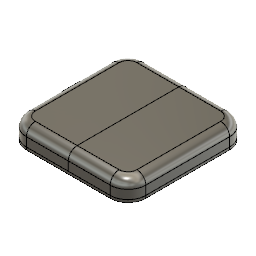
LightSwitch (Autodesk Fusion 360 design; units mm, degrees)
Autodesk Fusion 360 part; units mm, degrees
sketch "Sketch1" plane through (0, 0, 0) normal (0, 1, 0) x (1, 0, 0)
  line L0 (33.5, 33.5) -> (-33.5, -33.5) construction
  line L1 (-33.5, 33.5) -> (33.5, -33.5) construction
  line L2 (26.4289, -33.5) -> (33.5, -26.4289)
  line L3 (33.5, 26.4289) -> (26.4289, 33.5)
  line L4 (-26.4289, 33.5) -> (-33.5, 26.4289)
  line L5 (-33.5, -26.4289) -> (-26.4289, -33.5)
  line L6 (-33.5, 33.5) -> (-33.5, 26.4289)
  line L7 (-33.5, -26.4289) -> (-33.5, -33.5)
  line L8 (-33.5, 26.4289) -> (-33.5, -26.4289)
  line L9 (33.5, 33.5) -> (26.4289, 33.5)
  line L10 (-26.4289, 33.5) -> (-33.5, 33.5)
  line L11 (26.4289, 33.5) -> (-26.4289, 33.5)
  line L12 (-33.5, -33.5) -> (-26.4289, -33.5)
  line L13 (26.4289, -33.5) -> (33.5, -33.5)
  line L14 (-26.4289, -33.5) -> (26.4289, -33.5)
  line L15 (33.5, -33.5) -> (33.5, -26.4289)
  line L16 (33.5, 26.4289) -> (33.5, 33.5)
  line L17 (33.5, -26.4289) -> (33.5, 26.4289)
  line L18 (25.7919, 31.962) -> (-25.7919, 31.962)
  line L19 (-25.7919, 31.962) -> (-31.962, 25.7919)
  line L20 (-31.962, 25.7919) -> (-31.962, -25.7919)
  line L21 (-31.962, -25.7919) -> (-25.7919, -31.962)
  line L22 (-25.7919, -31.962) -> (25.7919, -31.962)
  line L23 (25.7919, -31.962) -> (31.962, -25.7919)
  line L24 (31.962, -25.7919) -> (31.962, 25.7919)
  line L25 (31.962, 25.7919) -> (25.7919, 31.962)
  dimension "d1" = 67
  dimension "d2" = 67
  dimension "d3" = 10
  dimension "d6" = 360
  dimension "d10" = 7.0711
  dimension "d11" = 1.538
extrude "Extrude1" add sketch "Sketch1" along normal blind 1.5 contours L2 L3 L4 L5 L8 L11 L14 L17 | L2 L13 L15 | L5 L7 L12 | L3 L9 L16 | L4 L6 L10 | L18 L19 L20 L21 L22 L23 L24 L25 makes body 1
extrude "Extrude2" add 1 faces at (8.8096, 1.5, 11.1667) along direction (0, 1, 0) blind 10 on bodies 1 bodies 1
delete_face "DeleteFace1" 1 faces at (-33.5, 3.8333, 28.786) on bodies 1
delete_face "DeleteFace2" 1 faces at (28.786, 3.8333, 33.5) on bodies 1
delete_face "DeleteFace3" 1 faces at (33.5, 3.8333, -28.786) on bodies 1
delete_face "DeleteFace4" 1 faces at (-28.786, 3.8333, -33.5) on bodies 1
fillet "Fillet1" radius 5 4 edges at (0, 11.5, 33.5) (-33.5, 11.5, 0) (0, 11.5, -33.5) (33.5, 11.5, 0) on bodies 1
fillet "Fillet1" radius 10 4 edges at (-33.5, 5.75, -33.5) (-33.5, 5.75, 33.5) (33.5, 5.75, 33.5) (33.5, 5.75, -33.5) on bodies 1
shell "Shell1" thickness 1.5 removed faces 0 bodies 1
ref_plane "WorkPlane1" through (29.9645, 1.5, -29.9645) normal (0, 1, 0) x (1, 0, 0)
split "Split1" by plane through (29.9645, 1.5, -29.9645) normal (0, 1, 0) bodies 1 makes body 2 at (7.8333, 11.5, 9.5)
sketch "Sketch3" plane through (0, 0, 0) normal (0, 0, 1) x (1, 0, 0)
  line L0 (31, 1.5) -> (31, 6.5)
  line L1 (32.5, 6.5) -> (25.4289, 6.5)
  line L2 (31, 1.5) -> (31, 3.5)
  line L3 (31, 3.5) -> (30, 3)
  line L4 (32.5, 1.5) -> (25.4289, 1.5)
  line L5 (31, 1.5) -> (29.9, 1.5)
  line L6 (29.4, 2) -> (29.4, 3.4501)
  line L7 (29.4, 3.4501) -> (29.4, 4)
  line L8 (29.4, 4) -> (30.5, 4)
  line L9 (30.5, 4) -> (29.4, 3.4501)
  line L10 (30, 2.5) -> (30, 3)
  line L11 (31, 1.5) -> (28.5, 1.5)
  line L12 (28.5, 4) -> (28.5, 2)
  arc A0 (29.4, 2) -> (29.9, 1.5) centre (29.9, 2) ccw
  line L13 (28, 1.5) -> (26.4, 1.5)
  arc A1 (28, 1.5) -> (28.5, 2) centre (28, 2) ccw
  line L14 (30, 2.5) -> (31, 1.7)
  line L15 (30.5, 4) -> (30.5, 4.5)
  line L16 (30.5, 4.5) -> (29.5, 5.5)
  line L17 (29.5, 5.5) -> (29, 5.5)
  line L18 (29, 5.5) -> (28.5, 4.5)
  line L19 (28.5, 4.5) -> (28.5, 4)
  dimension "d20" = 0.5
  dimension "d21" = 0.5
  measures "d20" radius of A0
  measures "d21" radius of A1
sketch "Tornillos" plane through (0, 0, 0) normal (0, 1, 0) x (1, 0, 0)
  line L0 (26.4289, 33.5) -> (-26.4289, 33.5)
  line L1 (-7.6716, 33.5) -> (8, 33.5)
  line L2 (0, 33.5) -> (0, 28.5)
  line L3 (1.75, 30) -> (-1.75, 30)
  line L4 (-3, 28.75) -> (-3, 28.25)
  line L5 (-1.75, 27) -> (1.75, 27)
  line L6 (3, 28.25) -> (3, 28.75)
  line L7 (10.2609, 33.6305) -> (-3, 27) construction
  line L8 (-3, 30) -> (3, 27) construction
  arc A0 (3, 28.75) -> (1.75, 30) centre (1.75, 28.75) ccw
  arc A1 (1.75, 27) -> (3, 28.25) centre (1.75, 28.25) ccw
  arc A2 (-3, 28.25) -> (-1.75, 27) centre (-1.75, 28.25) ccw
  arc A3 (-1.75, 30) -> (-3, 28.75) centre (-1.75, 28.75) ccw
  line L9 (0, 0) -> (9, 0)
  line L10 (-1.75, -27) -> (1.75, -27)
  arc A4 (-3, -28.75) -> (-1.75, -30) centre (-1.75, -28.75) ccw
  line L11 (-3, -28.75) -> (-3, -28.25)
  arc A5 (-1.75, -27) -> (-3, -28.25) centre (-1.75, -28.25) ccw
  line L12 (0, -33.5) -> (0, -28.5)
  line L13 (1.75, -30) -> (-1.75, -30)
  line L14 (3, -28.25) -> (3, -28.75)
  line L15 (-3, -30) -> (3, -27) construction
  arc A6 (1.75, -30) -> (3, -28.75) centre (1.75, -28.75) ccw
  arc A7 (3, -28.25) -> (1.75, -27) centre (1.75, -28.25) ccw
  line L16 (10.2609, -33.6305) -> (-3, -27) construction
  line L17 (33.5, -26.4289) -> (33.5, 26.4289)
  line L18 (33.5, -23.5) -> (33.5, 23.5)
  line L19 (32.5, 0) -> (25.4289, 0)
  line L20 (33.5, -7.15) -> (33.5, 7)
  line L21 (32.5, 0) -> (22.5, 0)
  circle A8 centre (22.5, 0) radius 1.75
  line L22 (0, 0) -> (0, 8)
  circle A9 centre (-22.5, 0) radius 1.75
  dimension "d33" = 6
  dimension "d34" = 3
  dimension "d35" = 1.25
  dimension "d36" = 5
  dimension "d37" = 3
  dimension "d38" = 10
  dimension "d39" = 3.5
  dimension "d43" = 4
  dimension "d44" = 10
  dimension "d45" = 3
  dimension "d46" = 3
  measures "d35" radius of A0
  measures "d37" distance of L3 L5
  measures "d39" diameter of A8
  measures "d44" distance of L11 L14
  measures "d45" distance of L10 L13
  measures "d46" distance of L14
extrude "Extrude7" cut sketch "Tornillos" along normal blind 10 contours L3 L4 L5 L6 A0 A1 A2 A3 | L10 A4 L11 A5 L13 L14 A6 A7 bodies 1
sketch "Sketch14" plane through (0, 1.5, 0) normal (0, 1, 0) x (-1, 0, 0)
  line L0 (1.75, -30) -> (-1.75, -30)
  arc A0 (-3, -28.75) -> (-1.75, -30) centre (-1.75, -28.75) ccw
  line L1 (-3, -28.75) -> (-3, -28.25)
  arc A1 (-1.75, -27) -> (-3, -28.25) centre (-1.75, -28.25) ccw
  line L2 (-1.75, -27) -> (1.75, -27)
  arc A2 (3, -28.25) -> (1.75, -27) centre (1.75, -28.25) ccw
  line L3 (3, -28.25) -> (3, -28.75)
  arc A3 (1.75, -30) -> (3, -28.75) centre (1.75, -28.75) ccw
  line L4 (-1.75, 30) -> (1.75, 30)
  arc A4 (3, 28.75) -> (1.75, 30) centre (1.75, 28.75) ccw
  line L5 (3, 28.75) -> (3, 28.25)
  arc A5 (1.75, 27) -> (3, 28.25) centre (1.75, 28.25) ccw
  line L6 (1.75, 27) -> (-1.75, 27)
  arc A6 (-3, 28.25) -> (-1.75, 27) centre (-1.75, 28.25) ccw
  line L7 (-3, 28.25) -> (-3, 28.75)
  arc A7 (-1.75, 30) -> (-3, 28.75) centre (-1.75, 28.75) ccw
  arc A8 (33.5, 23.5) -> (23.5, 33.5) centre (23.5, 23.5) ccw
  line L8 (23.5, 33.5) -> (-23.5, 33.5)
  arc A9 (-23.5, 33.5) -> (-33.5, 23.5) centre (-23.5, 23.5) ccw
  line L9 (-33.5, 23.5) -> (-33.5, -23.5)
  arc A10 (-33.5, -23.5) -> (-23.5, -33.5) centre (-23.5, -23.5) ccw
  line L10 (-23.5, -33.5) -> (23.5, -33.5)
  arc A11 (23.5, -33.5) -> (33.5, -23.5) centre (23.5, -23.5) ccw
  line L11 (33.5, -23.5) -> (33.5, 23.5)
  line L12 (33.5, -33.5) -> (-33.5, -33.5)
  line L13 (-1.75, 30) -> (1.75, 30)
  line L14 (1.75, 27) -> (-1.75, 27)
  line L15 (-3, 28.25) -> (-3, 28.75)
  line L16 (-33.5, 33.5) -> (33.5, 33.5)
  line L17 (33.5, 33.5) -> (33.5, -33.5)
  line L18 (3, 28.75) -> (3, 28.25)
  line L19 (-1.75, -27) -> (1.75, -27)
  line L20 (1.75, -30) -> (-1.75, -30)
  line L21 (-3, -28.75) -> (-3, -28.25)
  line L22 (30.9, -21) -> (29, -21)
  line L23 (30.9, 7.5) -> (29, 7.5)
  line L24 (-33.5, 33.5) -> (33.5, -33.5) construction
  line L25 (9.5, -22.5) -> (19.5, -22.5)
  line L26 (-9.5, -29.5) -> (-9.5, -22.5)
  line L27 (29, 7.5) -> (29, 21)
  line L28 (19.5, -29.5) -> (9.5, -29.5)
  line L29 (19.5, -22.5) -> (19.5, -29.5)
  line L30 (29, -21) -> (29, -7.5)
  line L31 (0, 0) -> (0, -4)
  line L32 (-19.5, -29.5) -> (-9.5, -29.5)
  line L33 (0, 0) -> (-9, 0)
  line L34 (-19.5, -22.5) -> (-19.5, -29.5)
  line L35 (29, -7.5) -> (30.9, -7.5)
  line L36 (-9.5, 22.5) -> (-19.5, 22.5)
  line L37 (-9.5, 29.5) -> (-9.5, 22.5)
  line L38 (-33.5, -33.5) -> (-33.5, 33.5)
  line L39 (30.9, -7.5) -> (30.9, -21)
  line L40 (33.5, 33.5) -> (-33.5, -33.5) construction
  line L41 (0, 0) -> (-4.5, 0)
  line L42 (-9.5, -22.5) -> (-19.5, -22.5)
  line L43 (9.5, -29.5) -> (9.5, -22.5)
  line L44 (-33.5, 23.5) -> (-33.5, -23.5)
  line L45 (-30.9, 21) -> (-29, 21)
  line L46 (33.5, -23.5) -> (33.5, 23.5)
  line L47 (-23.5, -33.5) -> (23.5, -33.5)
  line L48 (-19.5, 29.5) -> (-9.5, 29.5)
  arc A12 (1.75, 27) -> (3, 28.25) centre (1.75, 28.25) ccw
  arc A13 (-3, 28.25) -> (-1.75, 27) centre (-1.75, 28.25) ccw
  line L49 (19.5, 29.5) -> (9.5, 29.5)
  arc A14 (-3, -28.75) -> (-1.75, -30) centre (-1.75, -28.75) ccw
  line L50 (-30.9, 7.5) -> (-30.9, 21)
  line L51 (29, 21) -> (30.9, 21)
  arc A15 (1.75, -30) -> (3, -28.75) centre (1.75, -28.75) ccw
  arc A16 (3, 28.75) -> (1.75, 30) centre (1.75, 28.75) ccw
  arc A17 (-23.5, 33.5) -> (-33.5, 23.5) centre (-23.5, 23.5) ccw
  arc A18 (-33.5, -23.5) -> (-23.5, -33.5) centre (-23.5, -23.5) ccw
  arc A19 (-1.75, -27) -> (-3, -28.25) centre (-1.75, -28.25) ccw
  arc A20 (-1.75, 30) -> (-3, 28.75) centre (-1.75, 28.75) ccw
  arc A21 (3, -28.25) -> (1.75, -27) centre (1.75, -28.25) ccw
  arc A22 (23.5, -33.5) -> (33.5, -23.5) centre (23.5, -23.5) ccw
  line L52 (-19.5, 22.5) -> (-19.5, 29.5)
  line L53 (9.5, 22.5) -> (19.5, 22.5)
  circle A23 centre (22.5, 0) radius 1.75
  line L54 (9.5, 29.5) -> (9.5, 22.5)
  circle A24 centre (-22.5, 0) radius 1.75
  line L55 (19.5, 22.5) -> (19.5, 29.5)
  arc A25 (33.5, 23.5) -> (23.5, 33.5) centre (23.5, 23.5) ccw
  line L56 (30.9, 21) -> (30.9, 7.5)
  line L57 (23.5, 33.5) -> (-23.5, 33.5)
  line L58 (-29, -7.5) -> (-29, -21)
  line L59 (-29, -21) -> (-30.9, -21)
  line L60 (-29, 7.5) -> (-30.9, 7.5)
  line L61 (-29, 21) -> (-29, 7.5)
  line L62 (-30.9, -7.5) -> (-29, -7.5)
  line L63 (-30.9, -21) -> (-30.9, -7.5)
  line L64 (3, -28.25) -> (3, -28.75)
  dimension "d133" = 360
  dimension "d134" = 67
  dimension "d135" = 67
  dimension "d136" = 10
  dimension "d137" = 7
  dimension "d138" = 14
  dimension "d139" = 4
  dimension "d144" = 33.5
  dimension "d145" = 33.5
  measures "d138" distance of L17 L29
  measures "d139" distance of L12 L28
extrude "Extrude16" cut sketch "Sketch14" against normal blind 10 contours L25 L28 L29 L43 | L26 L32 L34 L42 | L36 L37 L48 L52 | L49 L53 L54 L55 bodies 1
sketch "Encajar" plane through (0, 1.5, 0) normal (0, 1, 0) x (-1, 0, 0)
  line L0 (1.75, -30) -> (-1.75, -30)
  arc A0 (-3, -28.75) -> (-1.75, -30) centre (-1.75, -28.75) ccw
  line L1 (-3, -28.75) -> (-3, -28.25)
  arc A1 (-1.75, -27) -> (-3, -28.25) centre (-1.75, -28.25) ccw
  line L2 (-1.75, -27) -> (1.75, -27)
  arc A2 (3, -28.25) -> (1.75, -27) centre (1.75, -28.25) ccw
  line L3 (3, -28.25) -> (3, -28.75)
  arc A3 (1.75, -30) -> (3, -28.75) centre (1.75, -28.75) ccw
  line L4 (-1.75, 30) -> (1.75, 30)
  arc A4 (3, 28.75) -> (1.75, 30) centre (1.75, 28.75) ccw
  line L5 (3, 28.75) -> (3, 28.25)
  arc A5 (1.75, 27) -> (3, 28.25) centre (1.75, 28.25) ccw
  line L6 (1.75, 27) -> (-1.75, 27)
  arc A6 (-3, 28.25) -> (-1.75, 27) centre (-1.75, 28.25) ccw
  line L7 (-3, 28.25) -> (-3, 28.75)
  arc A7 (-1.75, 30) -> (-3, 28.75) centre (-1.75, 28.75) ccw
  arc A8 (33.5, 23.5) -> (23.5, 33.5) centre (23.5, 23.5) ccw
  line L8 (23.5, 33.5) -> (-23.5, 33.5)
  arc A9 (-23.5, 33.5) -> (-33.5, 23.5) centre (-23.5, 23.5) ccw
  line L9 (-33.5, 23.5) -> (-33.5, -23.5)
  arc A10 (-33.5, -23.5) -> (-23.5, -33.5) centre (-23.5, -23.5) ccw
  line L10 (-23.5, -33.5) -> (23.5, -33.5)
  arc A11 (23.5, -33.5) -> (33.5, -23.5) centre (23.5, -23.5) ccw
  line L11 (33.5, -23.5) -> (33.5, 23.5)
  line L12 (-32.5, 32.5) -> (32.5, 32.5)
  line L13 (32.5, 32.5) -> (32.5, -32.5)
  line L14 (32.5, -32.5) -> (-32.5, -32.5)
  line L15 (-32.5, -32.5) -> (-32.5, 32.5)
  line L16 (-32.5, 32.5) -> (32.5, -32.5) construction
  line L17 (32.5, 32.5) -> (-32.5, -32.5) construction
  line L18 (18, -28.5) -> (4, -28.5)
  line L19 (4, -28.5) -> (4, -21.5)
  line L20 (4, -21.5) -> (18, -21.5)
  line L21 (18, -21.5) -> (18, -28.5)
  line L22 (0, 0) -> (-9, 0)
  line L23 (0, 0) -> (0, -5)
  line L24 (0, 0) -> (-4.5, 0)
  line L25 (-4, -21.5) -> (-18, -21.5)
  line L26 (-4, -28.5) -> (-4, -21.5)
  line L27 (-18, -28.5) -> (-4, -28.5)
  line L28 (-18, -21.5) -> (-18, -28.5)
  line L29 (-4, 21.5) -> (-18, 21.5)
  line L30 (-4, 28.5) -> (-4, 21.5)
  line L31 (-18, 28.5) -> (-4, 28.5)
  line L32 (-18, 21.5) -> (-18, 28.5)
  line L33 (4, 21.5) -> (18, 21.5)
  line L34 (4, 28.5) -> (4, 21.5)
  line L35 (18, 28.5) -> (4, 28.5)
  line L36 (18, 21.5) -> (18, 28.5)
  dimension "d47" = 65
  dimension "d48" = 65
  dimension "d49" = 14
  dimension "d50" = 7
  dimension "d51" = 14.5
  dimension "d52" = 4
  dimension "d54" = 360
  measures "d51" distance of L13 L21
  measures "d52" distance of L14 L18
extrude "Extrude8" [suppressed]
sketch "Agujeros" plane through (0, 1.5, 0) normal (0, 1, 0) x (-1, 0, 0)
  line L0 (1.75, -30) -> (-1.75, -30)
  arc A0 (-3, -28.75) -> (-1.75, -30) centre (-1.75, -28.75) ccw
  line L1 (-3, -28.75) -> (-3, -28.25)
  arc A1 (-1.75, -27) -> (-3, -28.25) centre (-1.75, -28.25) ccw
  line L2 (-1.75, -27) -> (1.75, -27)
  arc A2 (3, -28.25) -> (1.75, -27) centre (1.75, -28.25) ccw
  line L3 (3, -28.25) -> (3, -28.75)
  arc A3 (1.75, -30) -> (3, -28.75) centre (1.75, -28.75) ccw
  line L4 (-1.75, 30) -> (1.75, 30)
  arc A4 (3, 28.75) -> (1.75, 30) centre (1.75, 28.75) ccw
  line L5 (3, 28.75) -> (3, 28.25)
  arc A5 (1.75, 27) -> (3, 28.25) centre (1.75, 28.25) ccw
  line L6 (1.75, 27) -> (-1.75, 27)
  arc A6 (-3, 28.25) -> (-1.75, 27) centre (-1.75, 28.25) ccw
  line L7 (-3, 28.25) -> (-3, 28.75)
  arc A7 (-1.75, 30) -> (-3, 28.75) centre (-1.75, 28.75) ccw
  arc A8 (33.5, 23.5) -> (23.5, 33.5) centre (23.5, 23.5) ccw
  line L8 (23.5, 33.5) -> (-23.5, 33.5)
  arc A9 (-23.5, 33.5) -> (-33.5, 23.5) centre (-23.5, 23.5) ccw
  line L9 (-33.5, 23.5) -> (-33.5, -23.5)
  arc A10 (-33.5, -23.5) -> (-23.5, -33.5) centre (-23.5, -23.5) ccw
  line L10 (-23.5, -33.5) -> (23.5, -33.5)
  arc A11 (23.5, -33.5) -> (33.5, -23.5) centre (23.5, -23.5) ccw
  line L11 (33.5, -23.5) -> (33.5, 23.5)
  circle A12 centre (0, 0) radius 19
  dimension "d57" = 38
  measures "d57" diameter of A12
extrude "Extrude9" cut sketch "Agujeros" against normal blind 5 contours A12 bodies 1
sketch "Sketch9" plane through (0, 0, -33.5) normal (0, 0, -1) x (-1, 0, 0)
  line L0 (-23.5, 1.5) -> (23.5, 1.5)
  line L1 (23.5, 1.5) -> (23.5, 6.5)
  line L2 (23.5, 6.5) -> (-23.5, 6.5)
  line L3 (-23.5, 6.5) -> (-23.5, 1.5)
  line L4 (10.5, 6) -> (18.5, 6)
  line L5 (18.5, 6) -> (18.5, 10)
  line L6 (18.5, 10) -> (10.5, 10)
  line L7 (10.5, 10) -> (10.5, 6)
  line L8 (-23.5, 0) -> (23.5, 0)
  line L9 (33.5, 1.5) -> (33.5, 6.5)
  dimension "d64" = 8
  dimension "d65" = 4
  dimension "d66" = 6
  dimension "d67" = 15
  measures "d66" distance of L4 L8
  measures "d67" distance of L5 L9
split "Split2" by plane through (0, 0, 0) normal (1, 0, 0) bodies 2 makes body 3 at (9.5, 11.5, -7.8333)
sketch "Sketch11" plane through (0, 10, 0) normal (0, -1, 0) x (1, 0, 0)
  line L0 (0, -27.5) -> (0, 27.5)
  line L1 (0, 27.5) -> (-22.5, 27.5)
  arc A0 (-22.5, 27.5) -> (-27.5, 22.5) centre (-22.5, 22.5) ccw
  line L2 (-27.5, 22.5) -> (-27.5, -22.5)
  arc A1 (-27.5, -22.5) -> (-22.5, -27.5) centre (-22.5, -22.5) ccw
  line L3 (-22.5, -27.5) -> (-17.5, -27.5)
  line L4 (-17.5, -27.5) -> (-17.5, -31.0707)
  line L5 (-17.5, -31.0707) -> (-9.5, -31.0707)
  line L6 (-9.5, -31.0707) -> (-9.5, -27.5)
  line L7 (-9.5, -27.5) -> (0, -27.5)
  line L8 (-9, 5) -> (-19, 5)
  line L9 (-19, 5) -> (-19, -5)
  line L10 (-19, -5) -> (-9, -5)
  line L11 (-9, -5) -> (-9, 5)
  line L12 (-9, 5) -> (-19, -5) construction
  line L13 (-19, 5) -> (-9, -5) construction
  line L14 (-11.5, -2.5) -> (-16.5, -2.5)
  line L15 (-16.5, -2.5) -> (-16.5, 2.5)
  line L16 (-16.5, 2.5) -> (-11.5, 2.5)
  line L17 (-11.5, 2.5) -> (-11.5, -2.5)
  line L18 (-11.5, -2.5) -> (-16.5, 2.5) construction
  line L19 (-16.5, -2.5) -> (-11.5, 2.5) construction
  line L20 (-15, 2.5) -> (-13, 2.5)
  line L21 (-13, 2.5) -> (-13, 3.5)
  line L22 (-13, 3.5) -> (-15, 3.5)
  line L23 (-15, 3.5) -> (-15, 2.5)
  line L24 (-15, -2.5) -> (-13, -2.5)
  line L25 (-13, -2.5) -> (-13, -3.5)
  line L26 (-13, -3.5) -> (-15, -3.5)
  line L27 (-15, -3.5) -> (-15, -2.5)
  line L28 (0, 31) -> (0, 32.5)
  line L29 (0, 32.5) -> (-22.5, 32.5)
  arc A2 (-22.5, 32.5) -> (-32.5, 22.5) centre (-22.5, 22.5) ccw
  line L30 (-32.5, 22.5) -> (-32.5, -22.5)
  arc A3 (-32.5, -22.5) -> (-22.5, -32.5) centre (-22.5, -22.5) ccw
  line L31 (-22.5, -32.5) -> (0, -32.5)
  line L32 (0, -32.5) -> (0, -31)
  line L33 (0, -31) -> (-22.5, -31)
  arc A4 (-31, -22.5) -> (-22.5, -31) centre (-22.5, -22.5) ccw
  line L34 (-31, -22.5) -> (-31, 22.5)
  arc A5 (-22.5, 31) -> (-31, 22.5) centre (-22.5, 22.5) ccw
  line L35 (-22.5, 31) -> (0, 31)
  line L36 (0, -28.5) -> (0, 28.5)
  line L37 (0, 28.5) -> (-23.5, 28.5)
  arc A6 (-23.5, 28.5) -> (-28.5, 23.5) centre (-23.5, 23.5) ccw
  line L38 (-28.5, 23.5) -> (-28.5, -23.5)
  arc A7 (-28.5, -23.5) -> (-23.5, -28.5) centre (-23.5, -23.5) ccw
  line L39 (-23.5, -28.5) -> (0, -28.5)
  line L40 (0, 0) -> (-14, 0)
  dimension "d79" = 14
  dimension "d80" = 10
  dimension "d81" = 10
  dimension "d82" = 5
  dimension "d83" = 5
  dimension "d84" = 2
  dimension "d85" = 1
  dimension "d86" = 1.5
  dimension "d87" = 2
  dimension "d88" = 1
  dimension "d89" = 1.5
  measures "d79" distance of L40.start
  measures "d86" distance of L17 L21
  measures "d89" distance of L15 L27
extrude "Extrude11" add sketch "Sketch11" along normal blind 2 contours L14 L24 L25 L26 L27 | L16 L20 L21 L22 L23 bodies 2
ref_plane "WorkPlane2" through (-14, 9, 0) normal (0, 0, -1) x (1, 0, 0)
sketch "Sketch12" plane through (-15, 9, 0) normal (0, 0, -1) x (1, 0, 0)
  line L0 (15, -1) -> (-7.5, -1)
  line L1 (1, -1) -> (3, -1)
  line L2 (3.5, -0.5) -> (3.5, 1.5)
  line L3 (3, -1) -> (-1, -1)
  line L4 (3.5, 1.5) -> (2.7482, 1.7736)
  line L5 (3.5, 1.5) -> (2.5001, 1.5) construction
  line L6 (3.5, 1.5) -> (3.5, 2.5)
  line L7 (2.7482, 1.7736) -> (2.7482, 2.0736)
  line L8 (3.5, -1) -> (4.5, -1)
  line L9 (4.5, 0) -> (4.5, 2.2)
  line L10 (3.5, 2.5) -> (4.2, 2.5)
  line L11 (3.5, 2.5) -> (2.7482, 2.0736)
  arc A0 (4.5, 2.2) -> (4.2, 2.5) centre (4.2, 2.2) ccw
  line L12 (5.5, -1) -> (4.2, -1)
  arc A1 (4.5, 0) -> (5.5, -1) centre (5.5, 0) ccw
  arc A2 (3, -1) -> (3.5, -0.5) centre (3, -0.5) ccw
  line L13 (1, -1) -> (1, -0.3)
  line L14 (-1.5, -0.5) -> (-1.5, 1.5)
  arc A3 (-1.5, -0.5) -> (-1, -1) centre (-1, -0.5) ccw
  line L15 (-1.5, 1.5) -> (-0.7482, 1.7736)
  line L16 (-0.7482, 1.7736) -> (-0.7482, 2.0736)
  line L17 (-1.5, 2.5) -> (-0.7482, 2.0736)
  line L18 (-1.5, 1.5) -> (-1.5, 2.5)
  line L19 (-1.5, 2.5) -> (-2.2, 2.5)
  arc A4 (-2.2, 2.5) -> (-2.5, 2.2) centre (-2.2, 2.2) ccw
  line L20 (-2.5, 0) -> (-2.5, 2.2)
  arc A5 (-3.5, -1) -> (-2.5, 0) centre (-3.5, 0) ccw
  line L21 (-1.5, -1) -> (-2.5, -1)
  line L22 (15, 2.5) -> (15, 7.5)
  line L23 (15, 7.5) -> (-7.5, 7.5)
  line L24 (-7.5, 7.5) -> (-7.5, 2.5)
  line L25 (-7.5, 2.5) -> (15, 2.5)
  line L26 (1, -1) -> (1, 2.7)
  line L27 (1, -1) -> (15, -1)
  dimension "d93" = 2.5
  dimension "d94" = 2.5
  dimension "d95" = 160
  dimension "d96" = 0.8
  dimension "d97" = 0.3
  dimension "d99" = 1
  dimension "d100" = 1
  dimension "d101" = 2.2
  dimension "d102" = 3.5
  dimension "d103" = 0.3
  dimension "d104" = 1
  dimension "d105" = 0.5
  dimension "d148" = 14
  measures "d93" distance of origin
  measures "d95" angle of L4 L5
  measures "d103" radius of A0
  measures "d104" radius of A1
  measures "d105" radius of A2
  measures "d148" distance of origin
extrude "Extrude12" add sketch "Sketch12" along normal mid plane 3 contours L0 L2 L6 L8 L9 L10 A0 L12 A1 A2 L25 L27 | L4 L6 L7 L11 | L0 L14 A3 L18 L19 A4 L20 A5 L21 L25 | L15 L16 L17 L18 bodies 2
pattern_circular "C-Pattern2" count 4 over 360 about axis through (-14, 10, 0) along (0, -1, 0) of "Extrude12"
delete_body "RemoveBody2" bodies 3
mirror "Mirror2" about plane through (0, 0, 0) normal (1, 0, 0) of bodies 2 makes body 4
extrude "Extrude10" [suppressed]
sketch "Sketch13" plane through (0, 1.5, 0) normal (0, 1, 0) x (-1, 0, 0)
  circle A0 centre (0, 0) radius 19
  line L0 (1.75, -30) -> (-1.75, -30)
  arc A1 (-3, -28.75) -> (-1.75, -30) centre (-1.75, -28.75) ccw
  line L1 (-3, -28.75) -> (-3, -28.25)
  arc A2 (-1.75, -27) -> (-3, -28.25) centre (-1.75, -28.25) ccw
  line L2 (-1.75, -27) -> (1.75, -27)
  arc A3 (3, -28.25) -> (1.75, -27) centre (1.75, -28.25) ccw
  line L3 (3, -28.25) -> (3, -28.75)
  arc A4 (1.75, -30) -> (3, -28.75) centre (1.75, -28.75) ccw
  line L4 (-1.75, 30) -> (1.75, 30)
  arc A5 (3, 28.75) -> (1.75, 30) centre (1.75, 28.75) ccw
  line L5 (3, 28.75) -> (3, 28.25)
  arc A6 (1.75, 27) -> (3, 28.25) centre (1.75, 28.25) ccw
  line L6 (1.75, 27) -> (-1.75, 27)
  arc A7 (-3, 28.25) -> (-1.75, 27) centre (-1.75, 28.25) ccw
  line L7 (-3, 28.25) -> (-3, 28.75)
  arc A8 (-1.75, 30) -> (-3, 28.75) centre (-1.75, 28.75) ccw
  arc A9 (33.5, 23.5) -> (23.5, 33.5) centre (23.5, 23.5) ccw
  line L8 (23.5, 33.5) -> (-23.5, 33.5)
  arc A10 (-23.5, 33.5) -> (-33.5, 23.5) centre (-23.5, 23.5) ccw
  line L9 (-33.5, 23.5) -> (-33.5, -23.5)
  arc A11 (-33.5, -23.5) -> (-23.5, -33.5) centre (-23.5, -23.5) ccw
  line L10 (-23.5, -33.5) -> (23.5, -33.5)
  arc A12 (23.5, -33.5) -> (33.5, -23.5) centre (23.5, -23.5) ccw
  line L11 (33.5, -23.5) -> (33.5, 23.5)
  line L12 (-30.5, 21) -> (30.5, 21)
  line L13 (30.5, 21) -> (30.5, -22)
  line L14 (30.5, -21) -> (-30.5, -21)
  line L15 (-30.5, -22) -> (-30.5, 21)
  line L16 (-30.5, 21) -> (30.5, -21) construction
  line L17 (30.5, 21) -> (-30.5, -21) construction
  line L18 (28.5, 19) -> (-28.5, 19)
  line L19 (-28.5, 19) -> (-28.5, -22)
  line L20 (-28.5, -19) -> (28.5, -19)
  line L21 (28.5, -22) -> (28.5, 19)
  line L22 (28.5, 19) -> (-28.5, -19) construction
  line L23 (-28.5, 19) -> (28.5, -19) construction
  line L24 (31.5, 22) -> (-31.5, 22)
  line L25 (-31.5, 22) -> (-31.5, -22)
  line L26 (-31.5, -22) -> (31.5, -22)
  line L27 (31.5, -22) -> (31.5, 22)
  line L28 (31.5, 22) -> (-31.5, -22) construction
  line L29 (-31.5, 22) -> (31.5, -22) construction
  line L30 (30.5, -22) -> (31, -22) construction
  line L31 (30.5, -22) -> (29.3523, -20.6322)
  line L32 (30.5, -22) -> (31, -22) construction
  line L33 (29.4289, -20.4679) -> (30.5, -20.4679)
  line L34 (-30.5, -22) -> (-30.0866, -21.284)
  line L35 (-30.5, -22) -> (-29, -22) construction
  line L36 (-30.1732, -21.134) -> (-30, -21.134)
  arc A13 (-30.0866, -21.284) -> (-30.1732, -21.134) centre (-30.1732, -21.234) ccw
  arc A14 (29.4289, -20.4679) -> (29.3523, -20.6322) centre (29.4289, -20.5679) ccw
  line L37 (9.5, 29.5) -> (19.5, 29.5)
  line L38 (19.5, 29.5) -> (19.5, 22.5)
  line L39 (19.5, 22.5) -> (9.5, 22.5)
  line L40 (9.5, 22.5) -> (9.5, 29.5)
  line L41 (-19.5, -29.5) -> (-19.5, -22.5)
  line L42 (-19.5, -22.5) -> (-9.5, -22.5)
  line L43 (-9.5, -22.5) -> (-9.5, -29.5)
  line L44 (-9.5, -29.5) -> (-19.5, -29.5)
  line L45 (19.5, -22.5) -> (19.5, -29.5)
  line L46 (19.5, -29.5) -> (9.5, -29.5)
  line L47 (9.5, -29.5) -> (9.5, -22.5)
  line L48 (9.5, -22.5) -> (19.5, -22.5)
  line L49 (-9.5, 29.5) -> (-9.5, 22.5)
  line L50 (-9.5, 22.5) -> (-19.5, 22.5)
  line L51 (-19.5, 22.5) -> (-19.5, 29.5)
  line L52 (-19.5, 29.5) -> (-9.5, 29.5)
  dimension "d109" = 61
  dimension "d110" = 42
  dimension "d111" = 57
  dimension "d112" = 38
  dimension "d113" = 63
  dimension "d114" = 44
  dimension "d122" = 130
  dimension "d123" = 2
  dimension "d124" = 60
  dimension "d125" = 1
  dimension "d126" = 0.1
  dimension "d127" = 0.1
  measures "d122" angle of L31 L32
  measures "d124" angle of L34 L35
  measures "d126" radius of A13
  measures "d127" radius of A14
extrude "Extrude13" add sketch "Sketch13" along normal blind 2 contours L12 L13 L15 L24 L25 L26 L27 bodies 1
extrude "Extrude14" add sketch "Sketch13" along normal blind 1 from surface at 2 contours L12 L13 L14 L15 L18 L19 L21 L31 L33 A14 | L14 L15 L19 L26 | L14 L21 L26 L31 | L12 L13 L15 L24 L25 L26 L27 | L13 L14 L31 L33 A14 | L13 L14 L31 bodies 1
extrude "Extrude15" add sketch "Sketch13" along normal blind 1 from surface at 0.6 contours L13 L14 L31 L33 A14 | L13 L14 L31 bodies 1
fillet "Fillet2" radius 2 4 edges at (-28.5, 4, -22) (28.5, 4, -22) (-28.5, 4, 19) (28.5, 4, 19) on bodies 1
sketch "Sketch15" plane through (-33.5, 0, 0) normal (-1, 0, 0) x (0, 0, 1)
  line L0 (-23.5, 1.5) -> (23.5, 1.5)
  line L1 (23.5, 1.5) -> (23.5, 6.5)
  line L2 (23.5, 6.5) -> (-23.5, 6.5)
  line L3 (-23.5, 6.5) -> (-23.5, 1.5)
  line L4 (-5, 10) -> (5, 10)
  line L5 (5, 10) -> (5, 6)
  line L6 (5, 6) -> (-5, 6)
  line L7 (-5, 6) -> (-5, 10)
  line L8 (23.5, 11.5) -> (-23.5, 11.5)
  dimension "d149" = 10
  dimension "d150" = 4
  dimension "d151" = 5
  dimension "d152" = 1.5
  measures "d151" distance of origin L5
  measures "d152" distance of L4 L8
extrude "Extrude17" cut sketch "Sketch15" against normal blind 6 contours L2 L4 L5 L7 bodies 2
equation "d1 = d2"
equation "d46 = d33 / 2"
equation "d86 = d82 / 2 - 1 mm"
equation "d89 = d86"
equation "d95 = 180 deg - 20 deg"
equation "d111 = d109 - 4 mm"
equation "d112 = d110 - 4 mm"
equation "d113 = d109 + 2 mm"
equation "d114 = d110 + 2 mm"
equation "d124 = 90 deg - 30 deg"
equation "d144 = d135 / 2"
equation "d145 = d134 / 2"
equation "d151 = d149 / 2"
